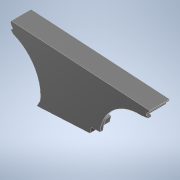
# Autodesk Inventor part: Pieza1_Carcasa
Saved by Autodesk Inventor 2022 (Build 260153000, 153)
## iProperties
Created: 2022-11-06
Part Number: Pieza1_Carcasa
Material: Resina acetálica, negra
Document SubType Name: Modeling
Designer: Mauricio Guerrero
Density: 1.425 g/cm^3
Appearance: Suave - Negro
Author: Mauricio Guerrero
## iProperties of the stored document Pieza1_Carcasa_3DPrint.ipt
Created: 2022-11-06
Part Number: Pieza1_Carcasa_3DPrint
Material: Genérico
Document SubType Name: Modeling
Designer: Mauricio Guerrero
Density: 1 g/cm^3
Appearance: Valor por defecto
Author: Mauricio Guerrero
Autodesk Inventor part; units mm, degrees
ref_plane "YZ Plane" through (0, 0, 0) normal (1, 0, 0) x (0, 1, 0)
ref_plane "XZ Plane" through (0, 0, 0) normal (0, 1, 0) x (-1, 0, 0)
ref_plane "XY Plane" through (0, 0, 0) normal (0, 0, 1) x (1, 0, 0)
sketch "Boceto1" plane through (0, 0, 0) normal (0, 0, 1) x (1, 0, 0)
  line L0 (42.8032, 3.438) -> (42.2388, 3.4264) construction
  line L1 (32.2478, 2.8886) -> (18.1678, 2.1307)
  line L2 (8.5818, 18.9887) -> (9.1664, 18.0334)
  line L3 (9.1664, 18.0334) -> (52.8836, 15.3138)
  arc A0 (54.0881, 17.2258) -> (54.0687, 17.2439) centre (52.0315, 15.0417) ccw
  line L4 (54.0687, 17.2439) -> (8.6649, 20.0685)
  line L5 (8.6649, 20.0685) -> (8.3833, 19.5786)
  line L6 (8.3833, 19.5786) -> (8.5818, 18.9887)
  line L7 (17.0583, 0.068) -> (31.7076, 0.8566)
  line L8 (17.0583, 0.068) -> (18.1678, 2.1307)
  arc A1 (53.8325, 16.6216) -> (52.8836, 15.3138) centre (54.4554, 15.1715) ccw
  line L9 (53.8325, 16.6216) -> (54.0881, 17.2258)
  line L10 (32.2478, 2.8886) -> (18.1678, 2.1307)
  line L11 (18.1678, 2.1307) -> (33.7743, 2.9708)
  line L12 (33.7743, 2.9708) -> (34.9191, 2.9708)
  line L13 (34.9191, 2.9708) -> (34.4156, 1.0024)
  line L14 (34.4156, 1.0024) -> (31.7076, 0.8566)
  point P0 (0, 0)
  point P1 (23.6867, 2.4277)
  point P2 (23.6867, 2.4277)
  point P3 (34.3467, 2.9708)
  dimension "d40" = 2
  dimension "d41" = 2
  constraints: 30 end point, 4 point on circle, 2 centre point, 1 horizontal, 1 midpoint, 4 other
  measures "d40" distance between parallel lines of L4 L3
  measures "d41" distance between parallel lines of L7 L10
extrude "Extrusión1" add sketch "Boceto1" against normal blind 6.5
sketch "Boceto2" plane through (0, 0, 0) normal (0, 0, 1) x (1, 0, 0)
  line L0 (8.9388, 9.1447) -> (47.9388, 9.1447) construction
  line L1 (51.4388, 12.1447) -> (51.4388, 15.3947) construction
  line L2 (9.1664, 16.6413) -> (8.4891, 17.498)
  line L3 (8.4891, 17.498) -> (9.1664, 18.0334)
  line L4 (9.1664, 18.0334) -> (52.8836, 15.3138)
  line L5 (33.7743, 2.9708) -> (18.1678, 2.1307) projected
  arc A0 (18.1678, 2.1307) -> (9.1664, 16.6413) centre (4.1736, 3.4968) ccw
  line L6 (18.1678, 2.1307) -> (33.7743, 2.9708)
  line L7 (33.7743, 2.9708) -> (37.722, 2.9708)
  arc A1 (51.2828, 14.4758) -> (37.722, 2.9708) centre (50.5158, 1.6354) ccw
  line L8 (52.8836, 15.3138) -> (53.5092, 15.187)
  line L9 (53.5092, 15.187) -> (53.4837, 14.7773)
  line L10 (53.4837, 14.7773) -> (51.2828, 14.4758)
  point P0 (0, 0)
  point P1 (1.4388, 9.1447)
  point P2 (23.6867, 2.4277)
  point P3 (51.9388, 13.5511)
  point P4 (32.2478, 2.8886)
  point P5 (40.9403, 9.1447)
  point P6 (32.2478, 2.8886)
  dimension "d27" = 3.5
  dimension "d31" = 3.25
  constraints: 20 end point, 4 point on circle, 2 centre point, 2 horizontal, 1 perpendicular, 1 point on line, 1 vertical
  measures "d27" horizontal distance of L0.end L1.start
  measures "d31" distance of L1.start L1.end
extrude "Extrusión2" add sketch "Boceto2" against normal blind 1
